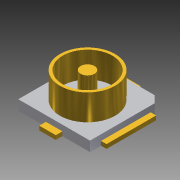
# Autodesk Inventor part: UMCC
Saved by Autodesk Inventor 2014 (Build 180170000, 170)
## iProperties
Created: 2015-11-06
Part Number: UMCC
Material: Generic
Document SubType Name: Modeling
Designer: Owner
Density: 1 g/cm^3
Appearance: Default
Author: Owner
Autodesk Inventor part; units mm, degrees
ref_plane "YZ Plane" through (0, 0, 0) normal (1, 0, 0) x (0, 1, 0)
ref_plane "XZ Plane" through (0, 0, 0) normal (0, 1, 0) x (-1, 0, 0)
ref_plane "XY Plane" through (0, 0, 0) normal (0, 0, 1) x (1, 0, 0)
sketch "Sketch1" plane through (0, 0, 0) normal (0, 1, 0) x (-1, 0, 0)
  line L0 (-1.493, 0.8155) -> (1.107, 0.8155)
  line L1 (1.107, 0.8155) -> (1.107, -1.7845)
  line L2 (1.107, -1.7845) -> (-1.2447, -1.7845)
  line L3 (-1.493, -1.5362) -> (-1.493, 0.8155)
  line L4 (-1.493, -1.5362) -> (-1.2447, -1.7845)
  point P0 (0, 0)
  dimension "d0" = 2.6
  dimension "d1" = 2.6
  constraints: 10 end point, 2 parallel, 1 horizontal, 1 perpendicular
  measures "d0" distance of L0.start L0.end
  measures "d1" distance of L0.end L1.end
extrude "Extrusion1" add sketch "Sketch1" along normal blind 0.36
sketch "Sketch2" plane through (0, 0.36, 0) normal (0, 1, 0) x (1, 0, 0)
  circle A0 centre (0.1676, 0.4207) radius 1
  circle A1 centre (0.1676, 0.4207) radius 0.25
  circle A2 centre (0.1676, 0.4207) radius 0.9
  point P0 (0, 0)
  dimension "d4" = 2
  dimension "d5" = 0.5
  dimension "d6" = 1.8
  constraints: 3 centre point, 2 coincident
  measures "d4" diameter of A0
  measures "d5" diameter of A1
  measures "d6" diameter of A2
extrude "Extrusion2" add sketch "Sketch2" along normal blind 0.94
sketch "Sketch3" plane through (0, 0, 0) normal (0, -1, 0) x (1, 0, 0)
  line L0 (1.493, 0.8155) -> (-1.107, 0.8155) projected
  line L1 (-1.107, 0.8155) -> (-1.107, -1.7845) projected
  line L2 (-1.107, -1.7845) -> (1.2447, -1.7845) projected
  line L3 (1.493, -1.5362) -> (1.493, 0.8155) projected
  line L4 (0.493, -2.0245) -> (-0.107, -2.0245)
  line L5 (-0.107, -2.0245) -> (-0.107, -1.7845)
  line L6 (0.493, -1.7845) -> (0.493, -2.0245)
  line L7 (-0.107, 1.0555) -> (0.493, 1.0555)
  line L8 (0.493, 1.0555) -> (0.493, 0.8155)
  line L9 (-0.107, 0.8155) -> (-0.107, 1.0555)
  line L10 (1.693, -1.3845) -> (1.493, -1.3845)
  line L11 (1.493, 0.4155) -> (1.693, 0.4155)
  line L12 (1.693, 0.4155) -> (1.693, -1.3845)
  line L13 (-1.307, -1.3845) -> (-1.107, -1.3845)
  line L14 (-1.107, 0.4155) -> (-1.307, 0.4155)
  line L15 (-1.307, 0.4155) -> (-1.307, -1.3845)
  line L16 (1.493, 0.4155) -> (1.493, -1.3845)
  line L17 (-1.107, 0.4155) -> (-1.107, -1.3845)
  line L18 (0.493, 0.8155) -> (-0.107, 0.8155)
  line L19 (0.493, -1.7845) -> (-0.107, -1.7845)
  point P0 (0, 0)
  dimension "d9" = 1.8
  dimension "d10" = 1.8
  dimension "d11" = 0.6
  dimension "d12" = 0.6
  dimension "d13" = 3.08
  dimension "d14" = 3
  dimension "d15" = 0.2
  dimension "d17" = 0.4
  dimension "d18" = 0.4
  dimension "d19" = 0.24
  dimension "d20" = 1
  dimension "d21" = 1
  constraints: 32 end point, 8 point on line, 4 horizontal, 4 parallel, 2 perpendicular, 2 vertical
  measures "d9" distance of L11.end L10.start
  measures "d10" distance of L14.end L13.start
  measures "d11" distance of L7.start L7.end
  measures "d12" distance of L4.start L4.end
  measures "d13" distance between parallel lines of L4 L7
  measures "d14" distance between parallel lines of L15 L12
  measures "d15" distance of L10.start L10.end
  measures "d17" distance between parallel lines of L0 L11
  measures "d18" distance between parallel lines of L0 L14
  measures "d19" distance between parallel lines of L7 L18
  measures "d20" distance between parallel lines of L3 L8
  measures "d21" distance between parallel lines of L1 L5
extrude "Extrusion3" add sketch "Sketch3" against normal blind 0.15
body "Solid1"
